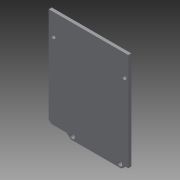
# Autodesk Inventor part: Arduino
Saved by Autodesk Inventor 2015 SP2 (Build 190223200, 223)
## iProperties
Created: 2016-09-02
Part Number: Arduino
Material: Generic
Document SubType Name: Modeling
Designer: jm799
Density: 1 g/cm^3
Appearance: Default
Author: jm799
Autodesk Inventor part; units mm, degrees
ref_plane "YZ Plane" through (0, 0, 0) normal (1, 0, 0) x (0, 1, 0)
ref_plane "XZ Plane" through (0, 0, 0) normal (0, 1, 0) x (-1, 0, 0)
ref_plane "XY Plane" through (0, 0, 0) normal (0, 0, 1) x (1, 0, 0)
sketch "Sketch1" plane through (0, 0, 0) normal (0, 1, 0) x (-1, 0, 0)
  line L0 (26.8759, 34.3) -> (-26.65, 34.3)
  line L1 (-25, -31.8) -> (-22, -34.3)
  line L2 (15, -31.8) -> (12, -34.3)
  line L3 (-25, -31.8) -> (-26.65, -31.8)
  line L4 (-22, -34.3) -> (12, -34.3)
  line L5 (-26.65, -31.8) -> (-26.65, 34.3)
  line L6 (25, -31.8) -> (26.8759, -30.2368)
  line L7 (25, -31.8) -> (15, -31.8)
  line L8 (26.8759, -30.2368) -> (26.8759, 34.3)
  line L9 (26.8759, 34.3) -> (-26.65, 34.3)
  line L10 (-26.65, -31.8) -> (-26.65, 34.3)
  line L11 (-26.65, -31.8) -> (-25, -31.8)
  line L12 (-25, -31.8) -> (-22, -34.3)
  line L13 (-22, -34.3) -> (12, -34.3)
  line L14 (12, -34.3) -> (15, -31.8)
  line L15 (15, -31.8) -> (25, -31.8)
  line L16 (25, -31.8) -> (26.8759, -30.2368)
  line L17 (26.8759, -30.2368) -> (26.8759, 34.3)
  point P0 (0, 0)
  point P1 (0, 0)
  constraints: 36 end point, 4 collinear, 4 parallel, 2 horizontal, 2 perpendicular, 1 coincident, 1 vertical
extrude "Extrusion1" add sketch "Sketch1" along normal blind 2
sketch "Sketch2" plane through (0, 2, 0) normal (0, 1, 0) x (1, 0, 0)
  line L0 (-26.8759, -34.3) -> (26.65, -34.3) construction
  line L1 (-24, -34.3) -> (-24, -20) construction
  circle A0 centre (-24, -20) radius 1.6
  line L2 (-0.1129, -34.3) -> (-0.1129, 34.3) construction
  line L3 (22, 34.3) -> (-12, 34.3) construction
  circle A1 centre (-24, -20) radius 1.6 construction
  circle A2 centre (23.7741, -20) radius 1.6
  point P0 (0, 0)
  dimension "d5" = 3.2
  constraints: 4 end point, 3 centre point, 2 coincident, 2 point on line, 2 vertical, 1 concentric, 1 midpoint, 1 symmetric about line, 1 other
  measures "d5" diameter of A0
sketch "Sketch3" plane through (0, 2, 0) normal (0, 1, 0) x (1, 0, 0)
  circle A0 centre (-11, 31.8) radius 1.6 construction
  circle A1 centre (-11, 31.8) radius 1.6
  circle A2 centre (21, 31.8) radius 1.6
  line L0 (-18, -34.3) -> (-18, -38) construction
  line L1 (-18, -38) -> (-8, -38) construction
  line L2 (-8, -38) -> (-8, -34.3) construction
  line L3 (24, -36) -> (16, -36) construction
  line L4 (16, -36) -> (16, -34.3) construction
  line L5 (24, -34.3) -> (24, -36)
  line L6 (16, -36) -> (16, -34.3)
  line L7 (-8, -34.3) -> (-8, -38)
  line L8 (-18, -38) -> (-18, -34.3)
  line L9 (-18, -38) -> (-8, -38)
  line L10 (16, -36) -> (24, -36)
  line L11 (-18, -34.3) -> (-8, -34.3)
  line L12 (-26.8759, -34.3) -> (26.65, -34.3) projected
  line L13 (16, -34.3) -> (24, -34.3)
  line L14 (-26.8759, -34.3) -> (26.65, -34.3)
  line L15 (26.65, -34.3) -> (24, -34.3)
  line L16 (24, -34.3) -> (24, -36)
  line L17 (24, -36) -> (16, -36)
  line L18 (16, -34.3) -> (-8, -34.3)
  line L19 (-8, -34.3) -> (-8, -38)
  line L20 (-18, -38) -> (-18, -34.3)
  line L21 (-26.8759, 30.2368) -> (-25, 31.8)
  line L22 (-25, 31.8) -> (-26.8759, 30.2368) projected
  line L23 (-15, 31.8) -> (-12, 34.3)
  line L24 (-12, 34.3) -> (-15, 31.8) projected
  line L25 (-12, 34.3) -> (22, 34.3)
  line L26 (22, 34.3) -> (-12, 34.3) projected
  line L27 (22, 34.3) -> (25, 31.8)
  line L28 (25, 31.8) -> (22, 34.3) projected
  line L29 (25, 31.8) -> (26.65, 31.8)
  line L30 (26.65, 31.8) -> (26.65, -34.3)
  line L31 (-26.8759, -34.3) -> (26.65, -34.3) projected
  line L32 (-11, 31.8) -> (21, 31.8) construction
  line L33 (5, 31.8) -> (5, 0) construction
  point P0 (0, 0)
  constraints: 56 end point, 14 collinear, 5 parallel, 3 centre point, 3 perpendicular, 2 vertical, 1 coincident, 1 concentric, 1 horizontal, 1 midpoint
hole "Hole1" at (-24, 2, 20) at (23.7741, 2, 20) direction (0, -1, 0) diameter 3.2 depth 8 tip angle 118
hole "Hole2" at (-11, 2, -31.8) at (21, 2, -31.8) direction (0, -1, 0) diameter 3.2 depth 8 tip angle 118
body "Solid1"
